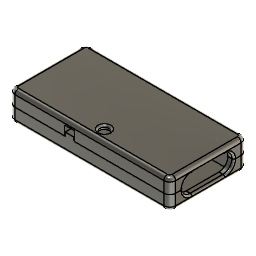
HIDman-mini (Autodesk Fusion 360 design; units mm, degrees)
Autodesk Fusion 360 part; units mm, degrees
note: some values were not read from the file. Set by a fixed rule: which sketch regions a step uses.
sketch "Sketch1" plane through (0, 0, 0) normal (0, 0, 1) x (1, 0, 0)
  line L0 (14, -9) -> (-14, -9)
  line L1 (-14, -9) -> (-14, 9)
  line L2 (-14, 9) -> (14, 9)
  line L3 (14, 9) -> (14, -9)
  line L4 (14, -9) -> (-14, 9) construction
  line L5 (-14, -9) -> (14, 9) construction
  line L6 (20.5, -9) -> (-20.5, -9)
  line L7 (-20.5, -9) -> (-20.5, 9)
  line L8 (-20.5, 9) -> (20.5, 9)
  line L9 (20.5, 9) -> (20.5, -9)
  line L10 (20.5, -9) -> (-20.5, 9) construction
  line L11 (-20.5, -9) -> (20.5, 9) construction
  line L12 (22.1, -10.6) -> (-22.1, -10.6)
  line L13 (-22.1, -10.6) -> (-22.1, 10.6)
  line L14 (-22.1, 10.6) -> (22.1, 10.6)
  line L15 (22.1, 10.6) -> (22.1, -10.6)
  line L16 (22.1, -10.6) -> (-22.1, 10.6) construction
  line L17 (-22.1, -10.6) -> (22.1, 10.6) construction
  line L18 (-5.9, -7) -> (-22.1, -7)
  line L19 (-22.1, -7) -> (-22.1, 7)
  line L20 (-22.1, 7) -> (-5.9, 7)
  line L21 (-5.9, 7) -> (-5.9, -7)
  line L22 (-5.9, -7) -> (-22.1, 7) construction
  line L23 (-22.1, -7) -> (-5.9, 7) construction
  circle A0 centre (1, -7.5) radius 1.3
  line L24 (-4.2, -10.6) -> (-6.8, -10.6)
  line L25 (-6.8, -10.6) -> (-6.8, -7.4)
  line L26 (-6.8, -7.4) -> (-4.2, -7.4)
  line L27 (-4.2, -7.4) -> (-4.2, -10.6)
  line L28 (-4.2, -10.6) -> (-6.8, -7.4) construction
  line L29 (-6.8, -10.6) -> (-4.2, -7.4) construction
  line L30 (20.4, -8.9) -> (-20.4, -8.9)
  line L31 (-20.4, -8.9) -> (-20.4, 8.9)
  line L32 (-20.4, 8.9) -> (20.4, 8.9)
  line L33 (20.4, 8.9) -> (20.4, -8.9)
  line L34 (20.4, -8.9) -> (-20.4, 8.9) construction
  line L35 (-20.4, -8.9) -> (20.4, 8.9) construction
  line L36 (-20.4, 8.9) -> (-14.9, 8.9)
  line L37 (-14.9, 8.9) -> (-14.9, 7)
  line L38 (-14.9, 7) -> (-20.4, 7)
  line L39 (-20.4, 7) -> (-20.4, 8.9)
  line L40 (-20.4, -8.9) -> (-14.9, -8.9)
  line L41 (-14.9, -8.9) -> (-14.9, -7)
  line L42 (-14.9, -7) -> (-20.4, -7)
  line L43 (-20.4, -7) -> (-20.4, -8.9)
  line L44 (20.4, 8.9) -> (14.9, 8.9)
  line L45 (14.9, 8.9) -> (14.9, 7)
  line L46 (14.9, 7) -> (20.4, 7)
  line L47 (20.4, 7) -> (20.4, 8.9)
  line L48 (20.4, -8.9) -> (14.9, -8.9)
  line L49 (14.9, -8.9) -> (14.9, -7)
  line L50 (14.9, -7) -> (20.4, -7)
  line L51 (20.4, -7) -> (20.4, -8.9)
  line L52 (14.9, 8.9) -> (14.9, 9)
  line L53 (20.4, 7) -> (20.5, 7)
  line L54 (20.4, -7) -> (20.5, -7)
  line L55 (14.9, -8.9) -> (14.9, -9)
  line L56 (-20.4, -7) -> (-20.5, -7)
  line L57 (-14.9, -8.9) -> (-14.9, -9)
  line L58 (-14.9, 8.9) -> (-14.9, 9)
  line L59 (-20.4, 7) -> (-20.5, 7)
  line L60 (-4.3, -10.6) -> (-6.7, -10.6)
  line L61 (-6.7, -10.6) -> (-6.7, -7.4)
  line L62 (-6.7, -7.4) -> (-4.3, -7.4)
  line L63 (-4.3, -7.4) -> (-4.3, -10.6)
  line L64 (-4.3, -10.6) -> (-6.7, -7.4) construction
  line L65 (-6.7, -10.6) -> (-4.3, -7.4) construction
  point P0 (-14, 0)
  point P1 (-14, 0)
  point P2 (-5.5, -9)
  point P3 (1, -7.5)
  point P4 (-5.5, -9)
  point P5 (-5.5, -9)
  dimension "d1" = 28
  dimension "d2" = 18
  dimension "d3" = 41
  dimension "d4" = 18
  dimension "d5" = 44.2
  dimension "d6" = 21.2
  dimension "d7" = 16.2
  dimension "d8" = 14
  dimension "d17" = 19.5
  dimension "d18" = 13
  dimension "d19" = 1.5
  dimension "d20" = 2.6
  dimension "d21" = 2.6
  dimension "d22" = 3.2
  dimension "d23" = 40.8
  dimension "d24" = 17.8
  dimension "d25" = 5.5
  dimension "d26" = 1.9
  dimension "d27" = 5.5
  dimension "d28" = 1.9
  dimension "d29" = 5.5
  dimension "d30" = 1.9
  dimension "d31" = 5.5
  dimension "d32" = 1.9
  dimension "d73" = 2.4
  dimension "d74" = 3.2
  constraint horizontal L0
  constraint perpendicular L0 L1
  constraint parallel L0 L2
  constraint parallel L1 L3
  constraint coincident L4 origin
  constraint coincident L5 origin
  constraint horizontal L6
  constraint perpendicular L6 L7
  constraint parallel L6 L8
  constraint parallel L7 L9
  constraint coincident L10 origin
  constraint coincident L11 origin
  constraint horizontal L12
  constraint perpendicular L12 L13
  constraint parallel L12 L14
  constraint parallel L13 L15
  constraint coincident L16 origin
  constraint coincident L17 origin
  constraint midpoint L1 P1
  constraint horizontal L18
  constraint perpendicular L18 L19
  constraint parallel L18 L20
  constraint parallel L19 L21
  constraint coincident L22 P1
  constraint coincident L23 P1
  constraint coincident P1 P0
  constraint coincident L6 P5
  constraint coincident P3 A0.centre
  constraint horizontal L24
  constraint perpendicular L24 L25
  constraint parallel L24 L26
  constraint parallel L25 L27
  constraint coincident L28 P5
  constraint coincident L29 P5
  constraint coincident P5 P4
  constraint horizontal L30
  constraint perpendicular L30 L31
  constraint parallel L30 L32
  constraint parallel L31 L33
  constraint coincident L34 origin
  constraint coincident L35 origin
  constraint horizontal L36
  constraint vertical L37
  constraint horizontal L38
  constraint vertical L39
  constraint horizontal L40
  constraint vertical L41
  constraint horizontal L42
  constraint vertical L43
  constraint horizontal L44
  constraint vertical L45
  constraint horizontal L46
  constraint vertical L47
  constraint horizontal L48
  constraint vertical L49
  constraint horizontal L50
  constraint vertical L51
  constraint coincident L8 L52.end
  constraint perpendicular L8 L52
  constraint coincident L9 L53.end
  constraint perpendicular L9 L53
  constraint coincident L9 L54.end
  constraint perpendicular L9 L54
  constraint coincident L6 L55.end
  constraint perpendicular L6 L55
  constraint coincident L7 L56.end
  constraint perpendicular L7 L56
  constraint coincident L6 L57.end
  constraint perpendicular L6 L57
  constraint coincident L8 L58.end
  constraint perpendicular L8 L58
  constraint coincident L7 L59.end
  constraint perpendicular L7 L59
  constraint horizontal L60
  constraint perpendicular L60 L61
  constraint parallel L60 L62
  constraint parallel L61 L63
  constraint coincident L64 P5
  constraint coincident L65 P5
  measures "d1" distance of L1.end L2.end
  measures "d2" distance of L0.end L1.end
  measures "d3" distance of L7.end L8.end
  measures "d4" distance of L6.end L7.end
  measures "d5" distance of L13.end L14.end
  measures "d6" distance of L12.end L13.end
  measures "d7" distance of L19.end L20.end
  measures "d8" distance of L18.end L19.end
  measures "d17" distance of L3 P5
  measures "d18" distance of L3 P3
  measures "d19" distance of L6 P3
  measures "d20" diameter of A0
  measures "d21" distance of L25.end L26.end
  measures "d22" distance of L24.end L25.end
  measures "d23" distance of L31.end L32.end
  measures "d24" distance of L30.end L31.end
  measures "d25" distance of L31.end L36.end
  measures "d26" distance of L31.end L38.end
  measures "d27" distance of L30.end L40.end
  measures "d28" distance of L30.end L42.end
  measures "d29" distance of L32.end L44.end
  measures "d30" distance of L32.end L46.end
  measures "d31" distance of L30.start L48.end
  measures "d32" distance of L30.start L50.end
  measures "d73" distance of L61.end L62.end
  measures "d74" distance of L60.end L61.end
extrude "Extrude1" add sketch "Sketch1" against normal blind 4 contours L0 L2 L6 L7 L8 L9 L12 L13 L14 L15 L20 L27 | L0 L6 L12 L24 L27 L63 | L6 L9 L30 L33 L48 L51 L54 L55 | L0 L6 L12 L24 L60 L61 L63 | L0 L6 L12 L24 L25 L61 | L8 L9 L32 L33 L44 L47 L52 L53 | L0 L6 L7 L12 L13 L18 L25 | L7 L8 L20 L31 L32 L36 L39 L58 L59 | L6 L7 L18 L30 L31 L40 L43 L56 L57 makes body 1
extrude "Extrude2" add sketch "Sketch1" against normal blind 1 from surface at -3 contours L0 L2 L6 L7 L8 L9 L12 L13 L14 L15 L20 L27 | L0 L3 L6 L27 L30 | L3 L6 L30 L55 | L0 L6 L27 L30 L63 | L1 L3 L18 L20 L21 L25 L26 L27 L30 L32 L62 | L3 L30 L32 L33 L45 L46 L49 L50 | L6 L9 L30 L33 L48 L51 L54 L55 | L0 L6 L30 L61 L63 | L26 L27 L30 L63 | L1 L2 L3 L8 L32 | L3 L8 L32 L52 | L30 L33 L48 L49 L50 L51 | L0 L6 L25 L30 L61 | L26 L30 L61 L62 L63 | L1 L8 L32 L58 | L1 L20 L32 L37 | L8 L9 L32 L33 L44 L47 L52 L53 | L32 L33 L44 L45 L46 L47 | L9 L33 L53 L54 | L0 L6 L7 L12 L13 L18 L25 | L0 L1 L6 L25 L30 | L25 L26 L30 L61 | L1 L18 L20 L21 | L1 L18 L20 L31 L38 L42 | L20 L31 L32 L36 L37 L38 L39 | L7 L8 L20 L31 L32 L36 L39 L58 L59 | L1 L6 L30 L57 | L1 L18 L30 L41 | L6 L7 L18 L30 L31 L40 L43 L56 L57 | L7 L13 L18 L19 L20 | L18 L30 L31 L40 L41 L42 L43 | L7 L18 L20 L31 L56 L59 | A0 bodies 1
extrude "Extrude3" add sketch "Sketch1" along normal blind 5.8 from surface at -3 contours L30 L33 L48 L49 L50 L51 | L32 L33 L44 L45 L46 L47 | L20 L31 L32 L36 L37 L38 L39 | L18 L30 L31 L40 L41 L42 L43 bodies 1
extrude "Extrude8" add sketch "Sketch1" along normal blind 1 contours L0 L6 L12 L24 L60 L61 L63 bodies 1
fillet "Fillet1" radius 1.6 4 edges at (-22.1, -10.6, -2) (22.1, -10.6, -2) (22.1, 10.6, -2) (-22.1, 10.6, -2) on bodies 1
fillet "Fillet1" radius 1 4 edges at (0, 10.6, -4) (-22.1, 0, -4) (22.1, 0, -4) (0, -10.6, -4) on bodies 1
extrude "Extrude4" add sketch "Sketch1" along normal blind 4 separate body contours L0 L2 L6 L7 L8 L9 L12 L13 L14 L15 L20 L27 | L0 L6 L12 L24 L27 L63 | L0 L6 L12 L24 L60 L61 L63 | L0 L6 L12 L24 L25 L61 | L0 L6 L7 L12 L13 L18 L25 makes body 2
extrude "Extrude5" add sketch "Sketch1" along normal blind 1 from surface at 3 contours L0 L3 L6 L27 L30 | L3 L6 L30 L55 | L0 L6 L27 L30 L63 | L1 L3 L18 L20 L21 L25 L26 L27 L30 L32 L62 | L3 L30 L32 L33 L45 L46 L49 L50 | L6 L9 L30 L33 L48 L51 L54 L55 | L0 L6 L30 L61 L63 | L26 L27 L30 L63 | L1 L2 L3 L8 L32 | L3 L8 L32 L52 | L30 L33 L48 L49 L50 L51 | L0 L6 L25 L30 L61 | L26 L30 L61 L62 L63 | L1 L8 L32 L58 | L1 L20 L32 L37 | L8 L9 L32 L33 L44 L47 L52 L53 | L32 L33 L44 L45 L46 L47 | L9 L33 L53 L54 | L0 L1 L6 L25 L30 | L25 L26 L30 L61 | L1 L18 L20 L21 | L1 L18 L20 L31 L38 L42 | L20 L31 L32 L36 L37 L38 L39 | L7 L8 L20 L31 L32 L36 L39 L58 L59 | L1 L6 L30 L57 | L1 L18 L30 L41 | L6 L7 L18 L30 L31 L40 L43 L56 L57 | L7 L13 L18 L19 L20 | L18 L30 L31 L40 L41 L42 L43 | L7 L18 L20 L31 L56 L59 bodies 2
extrude "Extrude6" cut sketch "Sketch1" along normal blind 2.6 contours L0 L6 L12 L24 L27 L63 | L0 L6 L12 L24 L60 L61 L63 | L0 L6 L12 L24 L25 L61 bodies 2
fillet "Fillet2" radius 1.6 4 edges at (22.1, -10.6, 2) (22.1, 10.6, 2) (-22.1, -10.6, 2) (-22.1, 10.6, 2) on bodies 2
fillet "Fillet2" radius 1 4 edges at (22.1, 0, 4) (0, -10.6, 4) (-22.1, 0, 4) (0, 10.6, 4) on bodies 2
fillet "Fillet2" radius 0.5 1 edges at (-0.212, -7.0299, 4) on bodies 2
sketch "Sketch2" plane through (22.1, 0, 0) normal (1, 0, 0) x (0, 1, 0)
  line L0 (-9, 0) -> (-9, -3)
  line L1 (-9, -3) -> (9, -3)
  line L2 (9, -3) -> (9, 0)
  line L3 (9, 0) -> (-9, 0)
  circle A0 centre (-4.5, 0) radius 2.5
  circle A1 centre (4.5, 0) radius 2.5
  line L4 (4.5, -2.5) -> (-4.5, -2.5)
  line L5 (-4.5, -2.5) -> (-4.5, 2.5)
  line L6 (-4.5, 2.5) -> (4.5, 2.5)
  line L7 (4.5, 2.5) -> (4.5, -2.5)
  line L8 (4.5, -2.5) -> (-4.5, 2.5) construction
  line L9 (-4.5, -2.5) -> (4.5, 2.5) construction
  point P0 (-4.5, 0)
  point P1 (4.5, 0)
  dimension "d57" = 4.5
  dimension "d58" = 4.5
  dimension "d59" = 5
  dimension "d60" = 5
  dimension "d63" = 9
  dimension "d64" = 5
  constraint coincident L3 P0
  constraint coincident L3 P1
  constraint coincident P0 A0.centre
  constraint coincident P1 A1.centre
  constraint horizontal L4
  constraint perpendicular L4 L5
  constraint parallel L4 L6
  constraint parallel L5 L7
  constraint coincident L8 origin
  constraint coincident L9 origin
  measures "d57" distance of origin A0.centre
  measures "d58" distance of origin P1
  measures "d59" diameter of A0
  measures "d60" diameter of A1
  measures "d63" distance of L5.end L6.end
  measures "d64" distance of L4.end L5.end
extrude "Extrude7" cut sketch "Sketch2" against normal blind 2 contours L3 A0 L5 | L3 A0 L5 | L3 A0 L5 | L3 A0 L5 | L3 A0 A1 L6 | L3 A0 A1 L4 | L3 A1 L7 | L3 A1 L7 | L3 A1 L7 | L3 A1 L7 bodies 1 2
fillet "Fillet3" radius 0.5 6 edges at (22.1, 6.2678, -1.7678) (22.1, 0, -2.5) (22.1, -6.2678, -1.7678) (22.1, -6.2678, 1.7678) (22.1, 0, 2.5) (22.1, 6.2678, 1.7678) on bodies 1 2
named bodies: "HIDman-mini_Base", "HIDman-mini_Top"
